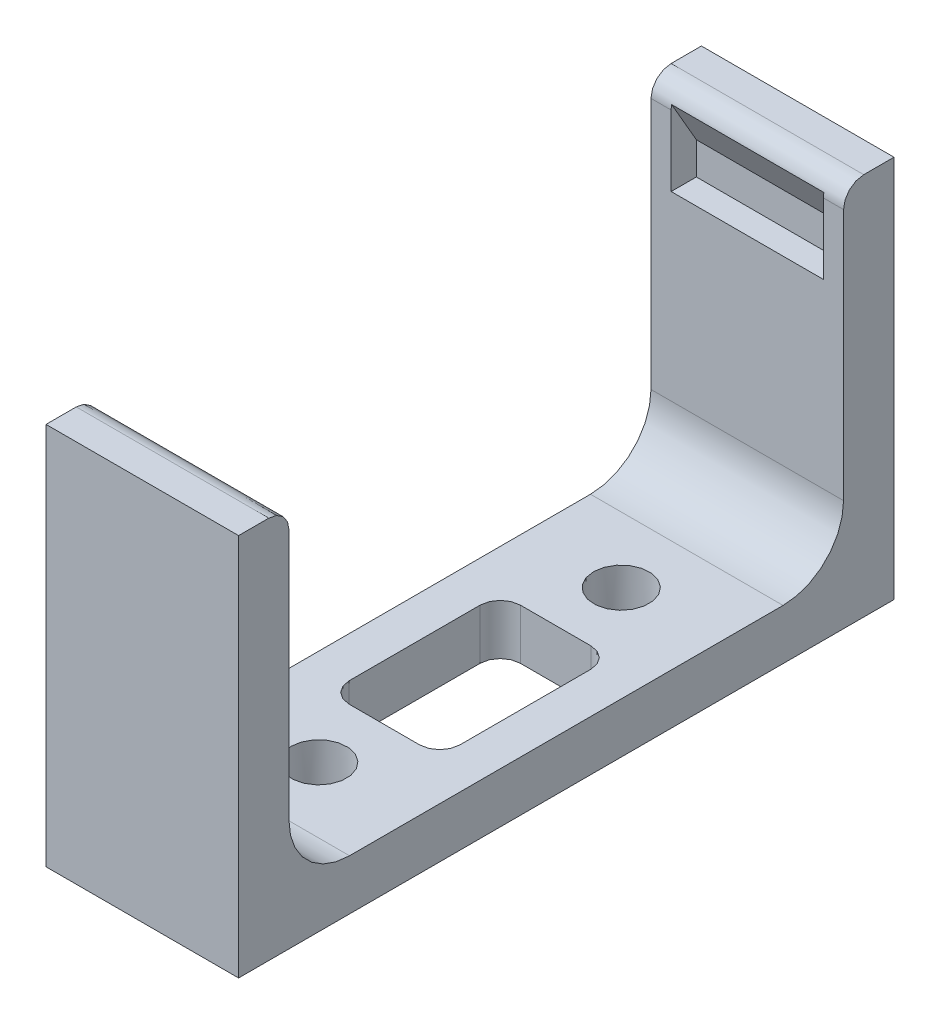
# Autodesk Inventor part: Base_Lower_v3
Saved by Autodesk Inventor 2021 (Build 250183000, 183)
## iProperties
Created: 2021-02-28
Part Number: Base_Lower_v3
Material: Generic
Document SubType Name: Modeling
Designer: Sam
Density: 1 g/cm^3
Appearance: Default
Author: Sam
Autodesk Inventor part; units mm, degrees
ref_plane "YZ Plane" through (0, 0, 0) normal (1, 0, 0) x (0, 1, 0)
ref_plane "XZ Plane" through (0, 0, 0) normal (0, 1, 0) x (-1, 0, 0)
ref_plane "XY Plane" through (0, 0, 0) normal (0, 0, 1) x (1, 0, 0)
sketch "Sketch1" plane through (0, 0, 0) normal (1, 0, 0) x (0, 1, 0)
  line L0 (38, 32.5) -> (0, 32.5)
  line L1 (0, 32.5) -> (0, -32.5)
  line L2 (0, -32.5) -> (38, -32.5)
  line L3 (0, 0) -> (16.8405, 0)
  line L4 (38, 32.5) -> (38, 27.5)
  line L5 (29, 27.5) -> (5, 27.5)
  line L6 (5, 27.5) -> (5, -27.5)
  line L7 (5, -27.5) -> (29, -27.5)
  line L8 (5.264, 15) -> (-3.604, 15) construction
  line L9 (5.264, -15) -> (-3.604, -15) construction
  line L10 (38, 27.5) -> (36.5301, 27.5)
  line L11 (29, 30) -> (29, 27.5)
  line L12 (36.5301, 27.5) -> (32.2, 30)
  line L13 (32.2, 30) -> (29, 30)
  line L14 (38, -32.5) -> (38, -27.5)
  line L15 (38, -27.5) -> (36.5301, -27.5)
  line L16 (29, -30) -> (29, -27.5)
  line L17 (36.5301, -27.5) -> (32.2, -30)
  line L18 (32.2, -30) -> (29, -30)
  dimension "d0" = 5
  dimension "d1" = 30
  dimension "d2" = 65
  dimension "d3" = 38
  dimension "d5" = 3.2
  dimension "d6" = 24
  dimension "d7" = 2.5
  dimension "d8" = 30
  dimension "d9" = 5
  dimension "d10" = 5
  dimension "d30" = 60
  constraints: 38 end point, 7 symmetric about line, 6 perpendicular, 5 horizontal, 1 midpoint, 1 vertical, 3 other
  measures "d0" distance between parallel lines of L1 L6
  measures "d1" distance between parallel lines of L9 L8
  measures "d2" distance of L0.end L1.end
  measures "d3" distance between parallel lines of L1 L4
  measures "d5" distance of L12.end L11.start
  measures "d6" distance between parallel lines of L6 L11
  measures "d7" distance of L11.start L5.start
  measures "d8" angle of L13 L12
  measures "d9" distance between parallel lines of L0 L5
  measures "d10" distance between parallel lines of L0 L10
  measures "d30" distance between parallel lines of L13 L18
extrude "Extrusion1" add sketch "Sketch1" along normal mid plane 15.1
sketch "Sketch2" plane through (7.55, 0, 0) normal (1, 0, 0) x (0, 0, -1)
  line L0 (32.5, 38) -> (27.5, 38) projected
  line L1 (27.5, 38) -> (27.5, 36.5301) projected
  line L2 (27.5, 36.5301) -> (30, 32.2) projected
  line L3 (30, 32.2) -> (30, 29) projected
  line L4 (30, 29) -> (27.5, 29) projected
  line L5 (27.5, 29) -> (27.5, 5) projected
  line L6 (27.5, 5) -> (-27.5, 5) projected
  line L7 (-27.5, 5) -> (-27.5, 29) projected
  line L8 (-27.5, 29) -> (-30, 29) projected
  line L9 (-30, 29) -> (-30, 32.2) projected
  line L10 (-30, 32.2) -> (-27.5, 36.5301) projected
  line L11 (-27.5, 36.5301) -> (-27.5, 38) projected
  line L12 (-27.5, 38) -> (-32.5, 38) projected
  line L13 (-32.5, 38) -> (-32.5, 0) projected
  line L14 (-32.5, 0) -> (32.5, 0) projected
  line L15 (32.5, 0) -> (32.5, 38) projected
  line L16 (-30, 32.2) -> (-27.5, 36.5301) projected
  line L17 (-27.5, 5) -> (-27.5, 29) projected
  line L18 (-27.5, 36.5301) -> (-27.5, 29)
  line L19 (27.5, 38) -> (27.5, 36.5301) projected
  line L20 (27.5, 29) -> (27.5, 5) projected
  line L21 (27.5, 36.5301) -> (27.5, 29)
  point P0 (0, 0)
  constraints: 4 end point, 2 collinear
extrude "Extrusion2" add sketch "Sketch2" along normal blind 2
mirror "Mirror1" about plane through (0, 0, 0) normal (1, 0, 0) of "Extrusion2"
fillet "Fillet1" radius 6 2 edges at (0, 5, 27.5) (0, 5, -27.5)
sketch "Sketch3" plane through (9.55, 0, -32.5) normal (0, -1, 0) x (1, 0, 0)
  line L0 (-9.55, 32.5) -> (28.6439, 32.5)
  point P0 (-9.55, 47.5)
  point P1 (-9.55, 17.5)
  dimension "d16" = 30
  constraints: 2 end point, 1 horizontal, 1 symmetric about line, 1 vertical alignment
  measures "d16" diameter of point (-9.55, 47.5) L0
hole "Hole1" at (0, 0, 15) at (0, 0, -15) direction (0, 1, 0) diameter 5.5 end through all
fillet "Fillet2" radius 2 2 edges at (0, 38, 27.5) (0, 38, -27.5)
sketch "Sketch4" plane through (-9.55, 5, -21.5) normal (0, 1, 0) x (1, 0, 0)
  line L0 (15.05, -13) -> (4.05, -13)
  line L1 (4.05, -13) -> (4.05, -30)
  line L2 (4.05, -30) -> (15.05, -30)
  line L3 (15.05, -30) -> (15.05, -13)
  point P0 (9.55, -21.5)
  point P1 (15.05, -21.5)
  point P2 (9.55, -13)
  dimension "d25" = 17
  dimension "d26" = 11
  constraints: 8 end point, 2 midpoint, 2 parallel, 1 horizontal, 1 horizontal alignment, 1 perpendicular, 1 vertical alignment
  measures "d25" distance of L2.end L0.start
  measures "d26" distance of L0.start L0.end
extrude "Extrusion3" cut sketch "Sketch4" against normal through all
fillet "Fillet3" radius 2 4 edges at (5.5, 2.5, -8.5) (-5.5, 2.5, -8.5) (-5.5, 2.5, 8.5) (5.5, 2.5, 8.5)
body "Solid1"
